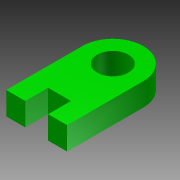
# Autodesk Inventor part: top_holder
Saved by Autodesk Inventor 2012 (Build 160160000, 160)
## iProperties
Created: 2013-10-02
Part Number: top_holder
Material: Default
Document SubType Name: Modeling
Designer: Nick
Density: 1 g/cm^3
Author: Nick
Autodesk Inventor part; units mm, degrees
ref_plane "YZ Plane" through (0, 0, 0) normal (1, 0, 0) x (0, 1, 0)
ref_plane "XZ Plane" through (0, 0, 0) normal (0, 1, 0) x (-1, 0, 0)
ref_plane "XY Plane" through (0, 0, 0) normal (0, 0, 1) x (1, 0, 0)
sketch "Sketch1" plane through (0, 0, 0) normal (0, 0, 1) x (1, 0, 0)
  line L0 (-1.5, -1.5) -> (-1.5, 1.5)
  line L1 (-1.5, 1.5) -> (1.5, 1.5)
  line L2 (1.5, 1.5) -> (1.5, -1.5)
  circle A0 centre (0, 8.5) radius 2.05
  line L3 (-1.5, -1.5) -> (1.5, 1.5) construction
  line L4 (1.5, -1.5) -> (-1.5, 1.5) construction
  circle A1 centre (0, 8.5) radius 4 construction
  arc A2 (4, 8.5) -> (-4, 8.5) centre (0, 8.5) ccw
  line L5 (-4, 8.5) -> (-4, -1.5)
  line L6 (4, 8.5) -> (4, -1.5)
  line L7 (-4, -1.5) -> (-1.5, -1.5)
  line L8 (1.5, -1.5) -> (4, -1.5)
  point P0 (0, 0)
  point P1 (0, 0)
  point P2 (0, 0)
  dimension "d0" = 4.1
  dimension "d1" = 3
  dimension "d3" = 3
  dimension "d4" = 3
  dimension "d5" = 10
  dimension "d6" = 8
  constraints: 18 end point, 4 point on circle, 4 tangent, 3 centre point, 3 equal length, 2 coincident, 2 midpoint, 2 perpendicular, 1 vertical, 1 vertical alignment
  measures "d0" diameter of A0
  measures "d1" distance between parallel lines of L2 L0
  measures "d3" distance of L1.end L2.end
  measures "d4" distance of L0.start L0.end
  measures "d5" vertical distance of A0.centre L2.end
  measures "d6" diameter of A1
extrude "Extrusion1" add sketch "Sketch1" along normal blind 3
body "Solid1"
